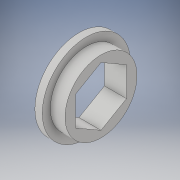
# Autodesk Inventor part: AxleBearingV1
Saved by Autodesk Inventor 2019 (Build 230136000, 136)
## iProperties
Created: 2021-09-16
Part Number: AxleBearingV1
Material: Generic
Document SubType Name: Modeling
Designer: timmy
Density: 1 g/cm^3
Appearance: Default
Author: timmy
Autodesk Inventor part; units mm, degrees
ref_plane "YZ Plane" through (0, 0, 0) normal (1, 0, 0) x (0, 1, 0)
ref_plane "XZ Plane" through (0, 0, 0) normal (0, 1, 0) x (-1, 0, 0)
ref_plane "XY Plane" through (0, 0, 0) normal (0, 0, 1) x (1, 0, 0)
sketch "Sketch1" plane through (0, 0, 0) normal (1, 0, 0) x (0, 1, 0)
  circle A0 centre (0, 0) radius 15.5575
  dimension "d0" = 31.115
  constraints: 1 centre point, 1 coincident
  measures "d0" diameter of A0
extrude "Extrusion1" add sketch "Sketch1" along normal blind 6.35
sketch "Sketch2" plane through (0, 0, 0) normal (-1, 0, 0) x (0, 0, 1)
  circle A0 centre (0, 0) radius 19.05
  dimension "d3" = 38.1
  constraints: 1 centre point, 1 coincident
  measures "d3" diameter of A0
extrude "Extrusion2" add sketch "Sketch2" along normal blind 3.175
sketch "Sketch3" plane through (6.35, 0, 0) normal (1, 0, 0) x (0, 0, -1)
  line L0 (0, 0) -> (0, 12.7)
  line L1 (0, 12.7) -> (10.9985, 6.35)
  line L2 (10.9985, 6.35) -> (10.9985, -6.35)
  line L3 (10.9985, -6.35) -> (0, -12.7)
  line L4 (0, -12.7) -> (-10.9985, -6.35)
  line L5 (-10.9985, -6.35) -> (-10.9985, 6.35)
  line L6 (-10.9985, 6.35) -> (0, 12.7)
  constraints: 14 end point, 1 coincident, 1 vertical, 13 other
extrude "Extrusion3" cut sketch "Sketch3" against normal up to surface (9.525 mm away)
body "Solid1"
